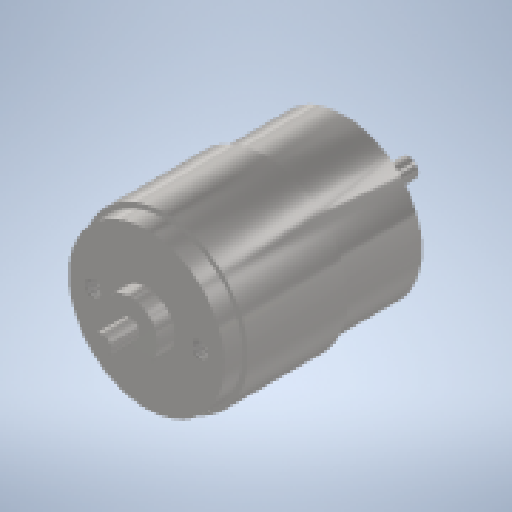
# Autodesk Inventor part: RZ735
Saved by Autodesk Inventor 2024 (Build 280153000, 153)
## iProperties
Created: 2023-05-29
Part Number: RZ735
Material: ステンレス鋼
Document SubType Name: Modeling
Designer: yuta2
Mass: 500 g
Surface Area: 114.448 cm^2
Volume: 81.5656 cm^3
Density: 6.13004 g/cm^3
Appearance: 半つや出し
Author: yuta2
Autodesk Inventor part; units mm, degrees
ref_plane "YZ Plane" through (0, 0, 0) normal (1, 0, 0) x (0, 1, 0)
ref_plane "XZ Plane" through (0, 0, 0) normal (0, 1, 0) x (-1, 0, 0)
ref_plane "XY Plane" through (0, 0, 0) normal (0, 0, 1) x (1, 0, 0)
sketch "スケッチ1" plane through (0, 0, 0) normal (1, 0, 0) x (0, 1, 0)
  line L0 (0, 0) -> (21.05, 0)
  line L1 (21.05, 0) -> (21.05, -53.5)
  line L2 (21.05, -53.5) -> (0, -53.5)
  line L3 (0, -53.5) -> (0, 0)
  line L4 (0, -53.5) -> (7.5, -53.5)
  line L5 (7.5, -53.5) -> (7.5, -57.8)
  line L6 (7.5, -57.8) -> (0, -57.8)
  line L7 (0, -57.8) -> (0, -53.5)
  line L8 (0, -57.8) -> (2.5, -57.8)
  line L9 (2.5, -57.8) -> (2.5, -71.1)
  line L10 (2.5, -71.1) -> (0, -71.1)
  line L11 (0, -71.1) -> (0, -57.8)
  line L12 (0, 0) -> (7.5, 0)
  line L13 (7.5, 0) -> (7.5, 4.4)
  line L14 (7.5, 4.4) -> (0, 4.4)
  line L15 (0, 4.4) -> (0, 0)
  line L16 (0, 4.4) -> (2.5, 4.4)
  line L17 (2.5, 4.4) -> (2.5, 11.9)
  line L18 (2.5, 11.9) -> (0, 11.9)
  line L19 (0, 11.9) -> (0, 4.4)
  line L20 (0, -4.9) -> (22.5, -4.9)
  line L21 (22.5, -4.9) -> (22.5, -31.9)
  line L22 (22.5, -31.9) -> (0, -31.9)
  line L23 (0, -31.9) -> (0, -4.9)
  point P0 (1.25, -71.1)
  point P1 (3.75, -53.5)
  point P2 (21.05, -4.9)
  point P3 (21.05, -31.9)
  dimension "d0" = 2.5
  dimension "d1" = 11.9
  dimension "d2" = 4.4
  dimension "d3" = 7.5
  dimension "d4" = 21.05
  dimension "d5" = 22.5
  dimension "d6" = 53.5
  dimension "d8" = 17.6
  dimension "d9" = 4.3
  dimension "d10" = 2.5
  dimension "d11" = 4.9
  dimension "d12" = 27
  constraints: 48 end point, 12 parallel, 6 horizontal, 6 perpendicular, 2 midpoint, 1 collinear, 1 point on line
  measures "d0" distance between parallel lines of L19 L17
  measures "d1" distance between parallel lines of L12 L18
  measures "d2" distance between parallel lines of L12 L14
  measures "d3" distance between parallel lines of L15 L13
  measures "d4" distance between parallel lines of L3 L1
  measures "d5" distance between parallel lines of L3 L21
  measures "d6" distance between parallel lines of L2 L0
  measures "d8" distance from line of point (1.25, -71.1) L2
  measures "d9" distance from line of point (3.75, -53.5) L6
  measures "d10" distance between parallel lines of L11 L9
  measures "d11" distance between parallel lines of L0 L20
  measures "d12" distance between parallel lines of L22 L20
revolve "回転1" add sketch "スケッチ1" angle 360 about axis through (0, 0, -31.9) along (0, 0, 1)
sketch "スケッチ2" plane through (0, 0, 0) normal (0, 0, 1) x (1, 0, 0)
  circle A0 centre (0, 0) radius 14.5
  point P0 (14.5, 0)
  point P1 (-14.5, 0)
  dimension "d14" = 29
  constraints: 2 horizontal alignment, 2 point on circle, 1 centre point, 1 coincident
  measures "d14" diameter of A0
hole "穴1" at (14.5, 0, 0) at (-14.5, 0, 0) direction (0, 0, -1) diameter 4 depth 8 tip angle 118
thread "ねじ1" size "M4x0.7" class "6H" standard "ANSI Metric M Profile" full length
thread "ねじ2" size "M4x0.7" class "6H" standard "ANSI Metric M Profile" full length
